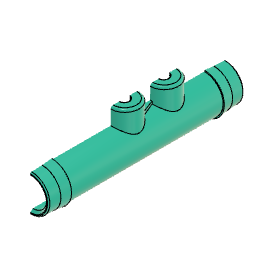
[Flow Measurement Venturi - 10-32 Style] v4 (Autodesk Fusion 360 design; units mm, degrees)
Autodesk Fusion 360 part; units mm, degrees
sketch "Sketch1" plane through (0, 0, 0) normal (0, 1, 0) x (1, 0, 0)
  circle A0 centre (0, 0) radius 11
  dimension "d1" = 22
  constraint coincident A0.centre origin
  measures "d1" diameter of A0
sketch "Sketch2" plane through (0, 0, 0) normal (1, 0, 0) x (0, 1, 0)
  line L0 (0, 0) -> (82.6556, 0) construction
  line L1 (82.1722, 7.7877) -> (77.6556, 7.9375)
  line L2 (5, 7.9375) -> (0.4834, 7.7877)
  line L3 (0, 7.2879) -> (0, 5.9375)
  line L4 (0, 5.9375) -> (45, 5.9375)
  line L5 (45, 5.9375) -> (53.5635, 2.8206)
  line L6 (54.2476, 2.7) -> (59.1199, 2.7)
  line L7 (59.4672, 2.7304) -> (77.6556, 5.9375)
  line L8 (77.6556, 5.9375) -> (82.6556, 5.9375)
  line L9 (82.6556, 7.2879) -> (82.6556, 5.9375)
  line L10 (0, 5.9375) -> (0, 0) construction
  line L11 (9, 7.9375) -> (73.6556, 7.9375)
  line L12 (82.6556, 0) -> (82.6556, 5.9375) construction
  arc A0 (53.5635, 2.8206) -> (54.2476, 2.7) centre (54.2476, 4.7) ccw
  arc A1 (59.1199, 2.7) -> (59.4672, 2.7304) centre (59.1199, 4.7) ccw
  arc A2 (0.4834, 7.7877) -> (0, 7.2879) centre (0.5, 7.2879) ccw
  arc A3 (82.6556, 7.2879) -> (82.1722, 7.7877) centre (82.1556, 7.2879) ccw
  line L13 (77.6556, 5.9375) -> (77.6556, 0) construction
  line L14 (45, 5.9375) -> (45, 0) construction
  line L15 (77.6556, 7.9375) -> (73.6556, 8.4375)
  line L16 (73.6556, 8.4375) -> (73.6556, 7.9375)
  line L17 (73.6556, 7.9375) -> (77.6556, 7.9375) construction
  line L18 (5, 7.9375) -> (9, 8.4375)
  line L19 (9, 8.4375) -> (9, 7.9375)
  line L20 (9, 7.9375) -> (5, 7.9375) construction
  point P0 (82.6556, 7.7716)
  point P1 (0, 7.7716)
  point P2 (53.8949, 2.7)
  point P3 (59.2949, 2.7)
  dimension "d60" = 20
  dimension "d61" = 2.7
  dimension "d62" = 5.4
  dimension "d63" = 10
  dimension "d66" = 2
  dimension "d67" = 2
  dimension "d68" = 0.5
  dimension "d69" = 0.5
  dimension "d72" = 5
  dimension "d74" = 2
  dimension "d75" = 1.9
  dimension "d77" = 5
  dimension "d78" = 1.9
  dimension "d81" = 7.9375
  dimension "d84" = 2
  dimension "d85" = 5.9375
  dimension "d94" = 4
  dimension "d95" = 0.5
  dimension "d96" = 0.5
  dimension "d97" = 4
  dimension "d105" = 45
  constraint coincident L0.start L10.end
  constraint horizontal L0
  constraint perpendicular L3 L4
  constraint perpendicular L3 L6
  constraint perpendicular L0 L10
  constraint vertical L9
  constraint horizontal L8
  constraint vertical L1.end L7.end
  constraint vertical L12
  constraint coincident P2 L5
  constraint coincident P2 L6
  constraint tangent L5 A0
  constraint tangent L6 A0
  constraint coincident P3 L6
  constraint coincident P3 L7
  constraint tangent L6 A1
  constraint tangent L7 A1
  constraint coincident P1 L2
  constraint coincident P1 L3
  constraint tangent L2 A2
  constraint tangent L3 A2
  constraint coincident P0 L1
  constraint coincident P0 L9
  constraint tangent L1 A3
  constraint tangent L9 A3
  constraint horizontal L11
  constraint coincident L0 L13.end
  constraint perpendicular L0 L13
  constraint coincident L0 L14.end
  constraint perpendicular L0 L14
  constraint perpendicular L11 L16
  constraint horizontal L17
  constraint perpendicular L11 L19
  constraint perpendicular L19 L20
  measures "d60" angle of L0 L5
  measures "d61" distance of L0 L6
  measures "d62" distance of P2 P3
  measures "d63" angle of L6 L7
  measures "d66" radius of A0
  measures "d67" radius of A1
  measures "d68" radius of A2
  measures "d69" radius of A3
  measures "d72" distance of L7.end L8.end
  measures "d74" distance of L1.end L7.end
  measures "d75" angle of L1 L8
  measures "d77" horizontal distance of L2.start L3.end
  measures "d78" angle of L2 L4
  measures "d81" distance of L0 L11
  measures "d84" distance of L4 L11
  measures "d85" distance of L0 L4
  measures "d94" distance of L1.end L16
  measures "d95" distance of L15.end L11.end
  measures "d96" distance of L18.end L11.start
  measures "d97" distance of L2.start L19
  measures "d105" distance of L3.end L4.end
sketch "Sketch14" plane through (0, 0, 0) normal (0, 0, 1) x (1, 0, 0)
  line L0 (0, 56.6838, 2.7) -> (9, 56.6838, 2.7)
  line L1 (0, 54.2476, 2.7) -> (0, 59.1199, 2.7)
revolve "Revolve1" add sketch "Sketch2" angle 360 about axis through (0, 0, 0) along (0, 1, 0)
ref_plane "WorkPlane1" through (0, 48.26, 0) normal (0, -1, 0) x (0, 0, -1)
sketch "Sketch4" plane through (0, 0, 0) normal (0, 0, 1) x (1, 0, 0)
  circle A0 centre (0, 56.6838) radius 1
  circle A1 centre (0, 40) radius 1
  line L0 (0, 56.6838) -> (9, 56.6838)
  dimension "d22" = 2
  dimension "d44" = 40
  constraint equal A0 A1
  constraint vertical origin A0.centre
  constraint vertical origin A1.centre
  constraint coincident A0.centre L0
  measures "d22" diameter of A0
  measures "d44" distance of origin A1.centre
extrude "Extrude1" cut sketch "Sketch4" along normal blind 12.7
ref_plane "WorkPlane2" through (0, 0, 4.445) normal (0, 0, 1) x (1, 0, 0)
sketch "Sketch5" plane through (0, 0, 4.445) normal (0, 0, 1) x (1, 0, 0)
ref_plane "WorkPlane3" through (0, 0, 15) normal (0, 0, 1) x (1, 0, 0)
sketch "Sketch9" plane through (0, 0, 15) normal (0, 0, 1) x (1, 0, 0)
  circle A0 centre (0, 56.6838) radius 6
  circle A1 centre (0, 40) radius 6
  circle A2 centre (0, 40) radius 1.5
  circle A3 centre (0, 56.6838) radius 1.5
  point P0 (0, 40)
  point P1 (0, 56.6838)
  dimension "d47" = 12
  dimension "d49" = 3
  dimension "d83" = 3
  constraint equal A0 A1
  constraint concentric A1 A2
  constraint concentric A0 A3
  constraint coincident P0 A1.centre
  constraint coincident A0.centre A3.centre
  measures "d47" diameter of A0
  measures "d49" diameter of A3
  measures "d83" diameter of A2
extrude "Extrude7" add sketch "Sketch9" along normal up to surface contours A0 end surface at (-1.8976, 40.9146, 7.7073)
sketch "Sketch10" plane through (0, 0, 0) normal (0, 0, 1) x (1, 0, 0)
sketch "Sketch11" plane through (0, 0, 0) normal (1, 0, 0) x (0, 1, 0)
sketch "Sketch12" plane through (0, 0, 0) normal (0, 1, 0) x (1, 0, 0)
sketch "Sketch13" plane through (0, 0, 0) normal (0, -1, 0) x (1, 0, 0)
  circle A0 centre (0, 0) radius 5.9375
  circle A1 centre (0, 0) radius 7.2879
extrude "Extrude9" add sketch "Sketch9" along normal up to surface contours A1 end surface at (-6.6087, 46.4715, 4.3964)
ref_plane "WorkPlane4" through (0, 19.2567, 7.9375) normal (0, 0, 1) x (-1, 0, 0)
sketch "Sketch15" plane through (0, 14.8767, 7.9375) normal (0, 0, 1) x (-1, 0, 0)
  line L0 (0, -38) -> (3, -30)
  line L1 (3, -30) -> (-3, -30)
  line L2 (-3, -30) -> (0, -38)
  line L3 (0, -38) -> (0, -30)
  line L4 (0, 5.8767) -> (0, -58.7789)
  circle A0 centre (0, -41.8071) radius 6
  circle A1 centre (0, -25.1233) radius 6
  constraint horizontal L1
  constraint coincident L1 L3.end
  constraint midpoint L1 L3.end
  constraint coincident L0.start L4
  constraint coincident L3.end L4
extrude "Extrude10" add sketch "Sketch15" along normal blind 1 and the other way blind 1 contours L0 L3 L4 A0 | L2 L3 L4 A0 | L0 L3 L4 A0 A1 | L2 L3 L4 A0 A1 | L0 L1 L3 L4 A1 | L1 L2 L3 L4 A1
hole "Hole1" at (0, 56.6838, 15) direction (0, 0, -1) diameter 4.064 depth 7 tip angle 180
thread "Thread1" "ANSI Unified Screw Threads 0.19(#10) 10-32 UNF 2B" major diameter 4.826 minor diameter 4.064 pitch 0.7937 angle 60 modelled right hand crest width 0.2253 on face at (0.2023, 54.6619, 12.6667) crest through (2.032, 56.6838, 14.8016)
hole "Hole2" at (0, 40, 15) direction (0, 0, -1) diameter 4.064 depth 7 tip angle 180
thread "Thread2" "ANSI Unified Screw Threads 0.19(#10) 10-32 UNF 2B" major diameter 4.826 minor diameter 4.064 pitch 0.7937 angle 60 modelled right hand crest width 0.2253 on face at (0.2023, 37.9781, 12.6667) crest through (2.032, 40, 14.8016)
fillet "Fillet1" radius 1 2 edges at (-5.594, 54.5141, 15) (-5.594, 37.8303, 15)
chamfer "Chamfer1" distance 1 angle 45 1 edges at (-5.5357, 0, 2.1471)
equation "d61 = ( 5.4 / 2 ) * 1 mm"
equation "d62 = d61 * 2"
equation "d83 = d49"
